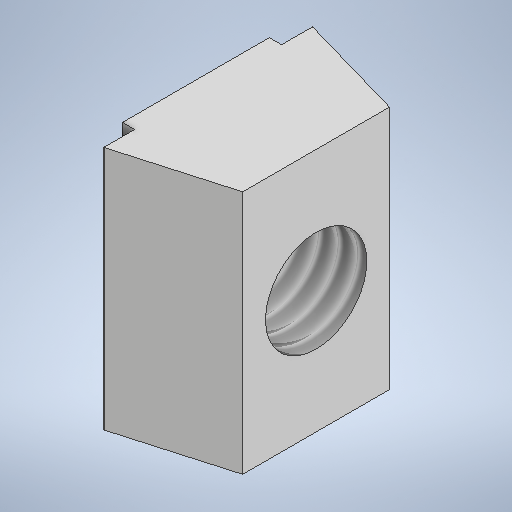
# Autodesk Inventor part: m5_t_nut
Saved by Autodesk Inventor 2025 (Build 290162000, 162)
## iProperties
Created: 2026-06-24
Part Number: m5_t_nut
Material: Generic
Document SubType Name: Modeling
Designer: localadmin
Density: 1 g/cm^3
Appearance: Default
Author: localadmin
Autodesk Inventor part; units mm, degrees
ref_plane "YZ Plane" through (0, 0, 0) normal (1, 0, 0) x (0, 1, 0)
ref_plane "XZ Plane" through (0, 0, 0) normal (0, 1, 0) x (-1, 0, 0)
ref_plane "XY Plane" through (0, 0, 0) normal (0, 0, 1) x (1, 0, 0)
sketch "Sketch1" plane through (0, 0, 0) normal (0, 1, 0) x (-1, 0, 0)
  line L0 (0, -3) -> (-0.5, -3)
  line L1 (-0.5, -3) -> (-0.5, -4.2634)
  line L2 (-0.5, -4.2634) -> (-0.5134, -4.2634)
  line L3 (-0.5134, -4.2634) -> (-4.9134, -3)
  line L4 (0, -3) -> (0, 0)
  line L5 (-4.9134, -3) -> (-4.9134, 0)
  line L6 (0, 0) -> (-4.9134, 0) construction
  line L7 (0, 3) -> (-0.5, 3)
  line L8 (-0.5, 3) -> (-0.5, 4.2634)
  line L9 (-0.5, 4.2634) -> (-0.5134, 4.2634)
  line L10 (-0.5134, 4.2634) -> (-4.9134, 3)
  line L11 (0, 3) -> (0, 0)
  line L12 (-4.9134, 3) -> (-4.9134, 0)
  dimension "d0" = 6
  dimension "d1" = 0.5
  dimension "d4" = 4.4
  constraints: 26 end point, 5 symmetric about line, 2 perpendicular, 2 point on line, 2 vertical, 1 horizontal
  measures "d0" distance of L0.start L11.start
  measures "d1" distance of L0.end L0.start
  measures "d4" horizontal distance of L2.end L3.end
extrude "Extrusion1" add sketch "Sketch1" along normal blind 10
sketch "Sketch2" plane through (0, 0, -3) normal (-1, 0, 0) x (0, 0, 1)
  line L0 (3, 0) -> (3, 10) construction
  line L1 (0, 10) -> (6, 10) projected
  point P0 (3, 5)
  constraints: 2 end point, 2 midpoint
hole "Hole2" at (0, 5, 0) direction (1, 0, 0) diameter 4.134 end through all thread size "M5x0.8" class "6H" standard "ISO Metric profile"
body "Solid1"
